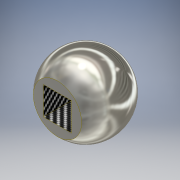
# Autodesk Inventor part: Femoral Head DP-2
Saved by Autodesk Inventor 2018 (Build 220112000, 112)
## iProperties
Created: 2018-11-23
Part Number: Femoral Head DP-2
Material: Silver
Document SubType Name: Modeling
Designer: Ousama
Density: 10.49 g/cm^3
Appearance: Silver
Mass: 280.059 g
Surface Area: 60.5414 cm^2
Volume: 26.6977 cm^3
Author: Ousama
Autodesk Inventor part; units mm, degrees
ref_plane "YZ Plane" through (0, 0, 0) normal (1, 0, 0) x (0, 1, 0)
ref_plane "XY Plane" through (0, 0, 0) normal (0, 0, 1) x (1, 0, 0)
sketch "Sketch1" plane through (0, 0, 0) normal (0, 0, 1) x (1, 0, 0)
  arc A0 (0, -19.8) -> (0, 19.8) centre (0, 0) ccw
  line L0 (0, 19.8) -> (0, -19.8)
  dimension "d0" = 19.8
  constraints: 2 end point, 2 point on circle, 1 centre point, 1 coincident, 1 vertical
  measures "d0" radius of A0
revolve "Revolution1" add sketch "Sketch1" angle 360 about axis through (0, 19.8, 0) along (0, -1, 0)
ref_plane "Work Plane1" through (0, -15, 0) normal (0, 1, 0) x (-1, 0, 0)
split_face "Split1"
split "Split2" plane through (0, -15, 0) removes the side toward (0, -1, 0)
sketch "Sketch3" plane through (0, -15, 0) normal (0, 1, 0) x (-1, 0, 0)
  line L0 (-7.5, -7.5) -> (7.5, -7.5)
  line L1 (7.5, -7.5) -> (7.5, 7.5)
  line L2 (7.5, 7.5) -> (-7.5, 7.5)
  line L3 (-7.5, 7.5) -> (-7.5, -7.5)
  line L4 (-7.5, -7.5) -> (7.5, 7.5) construction
  line L5 (7.5, -7.5) -> (-7.5, 7.5) construction
  point P0 (0, 0)
  dimension "d10" = 15
  dimension "d11" = 15
  constraints: 12 end point, 2 midpoint, 2 parallel, 1 horizontal, 1 perpendicular
  measures "d10" distance of L2.end L1.end
  measures "d11" distance of L1.end L0.end
extrude "Extrusion1" cut sketch "Sketch3" along normal blind 20
body "Solid1"
